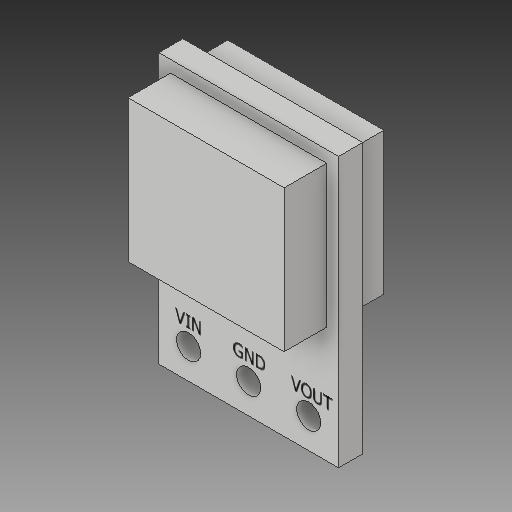
# Autodesk Inventor part: S7V7F5
Saved by Autodesk Inventor 2018 (Build 220112000, 112)
## iProperties
Part Number: S7V7F5
Material: 一般
Document SubType Name: Modeling
Designer: sktom
Density: 1 g/cm^3
Appearance: 既定
Author: sktom
Autodesk Inventor part; units mm, degrees
ref_plane "YZ Plane" through (0, 0, 0) normal (1, 0, 0) x (0, 1, 0)
ref_plane "XZ Plane" through (0, 0, 0) normal (0, 1, 0) x (-1, 0, 0)
ref_plane "XY Plane" through (0, 0, 0) normal (0, 0, 1) x (1, 0, 0)
sketch "スケッチ1" plane through (0, 0, 0) normal (0, 0, 1) x (1, 0, 0)
  line L0 (-3.8, -5.7) -> (3.8, -5.7)
  line L1 (3.8, -5.7) -> (3.8, 5.7)
  line L2 (3.8, 5.7) -> (-3.8, 5.7)
  line L3 (-3.8, 5.7) -> (-3.8, -5.7)
  line L4 (-3.8, -5.7) -> (3.8, 5.7) construction
  line L5 (3.8, -5.7) -> (-3.8, 5.7) construction
  circle A0 centre (0, -4.43) radius 0.51
  circle A1 centre (-2.54, -4.43) radius 0.51
  circle A2 centre (2.54, -4.43) radius 0.51
  point P0 (0, 0)
  point P1 (0, 0)
  dimension "d0" = 11.4
  dimension "d1" = 7.6
  dimension "d2" = 1.27
  dimension "d3" = 2.54
  dimension "d4" = 2.54
  dimension "d5" = 1.02
  constraints: 12 end point, 3 centre point, 3 midpoint, 2 equal radius, 2 horizontal alignment, 2 parallel, 1 horizontal, 1 perpendicular, 1 vertical alignment
  measures "d0" distance of L0.end L1.end
  measures "d1" distance of L1.end L2.end
  measures "d2" distance from line of L0 A2.centre
  measures "d3" distance of A2.centre A0.centre
  measures "d4" distance of A0.centre A1.centre
  measures "d5" diameter of A1
extrude "押し出し1" add sketch "スケッチ1" along normal blind 1.02
sketch "スケッチ2" plane through (0, 0, 1.02) normal (0, 0, 1) x (1, 0, 0)
  line L0 (-3.3, 5.2) -> (3.3, 5.2)
  line L1 (3.3, 5.2) -> (3.3, -0.8)
  line L2 (3.3, -0.8) -> (-3.3, -0.8)
  line L3 (-3.3, -0.8) -> (-3.3, 5.2)
  line L4 (-3.3, 5.2) -> (3.3, -0.8) construction
  line L5 (3.3, 5.2) -> (-3.3, -0.8) construction
  line L6 (3.8, 5.7) -> (-3.8, 5.7) projected
  line L7 (-3.8, 5.7) -> (-3.8, -5.7) projected
  line L8 (3.8, -5.7) -> (3.8, 5.7) projected
  point P0 (0, 0)
  point P1 (0, 2.2)
  dimension "d8" = 0.5
  dimension "d9" = 0.5
  dimension "d10" = 0.5
  dimension "d11" = 6
  constraints: 12 end point, 2 midpoint, 2 parallel, 1 horizontal, 1 perpendicular
  measures "d8" distance between parallel lines of L6 L0
  measures "d9" distance between parallel lines of L7 L3
  measures "d10" distance between parallel lines of L8 L1
  measures "d11" distance of L0.end L1.end
extrude "押し出し2" add sketch "スケッチ2" along normal blind 1.8
sketch "スケッチ3" plane through (0, 0, 0) normal (0, 0, -1) x (-1, 0, 0)
  line L0 (-3.3, 5.2) -> (3.3, 5.2) projected
  line L1 (3.3, 5.2) -> (3.3, -0.8) projected
  line L2 (3.3, -0.8) -> (-3.3, -0.8) projected
  line L3 (-3.3, -0.8) -> (-3.3, 5.2) projected
  point P0 (0, 0)
extrude "押し出し3" add sketch "スケッチ3" along normal blind 1.4
sketch "スケッチ4" plane through (0, 0, 1.02) normal (0, 0, 1) x (1, 0, 0)
  line L0 (-3.0991, -3.2712) -> (-1.8939, -3.2712) construction
  line L1 (-1.8939, -3.2712) -> (-1.8939, -3.8169) construction
  line L2 (-1.8939, -3.8169) -> (-3.0991, -3.8169) construction
  line L3 (-3.0991, -3.8169) -> (-3.0991, -3.2712) construction
  line L4 (-0.6641, -3.2466) -> (0.9346, -3.2466) construction
  line L5 (0.9346, -3.2466) -> (0.9346, -3.8169) construction
  line L6 (0.9346, -3.8169) -> (-0.6641, -3.8169) construction
  line L7 (-0.6641, -3.8169) -> (-0.6641, -3.2466) construction
  line L8 (1.7955, -3.2958) -> (3.5455, -3.2958) construction
  line L9 (3.5455, -3.2958) -> (3.5455, -3.8169) construction
  line L10 (3.5455, -3.8169) -> (1.7955, -3.8169) construction
  line L11 (1.7955, -3.8169) -> (1.7955, -3.2958) construction
  point P0 (0, 0)
  constraints: 6 other
